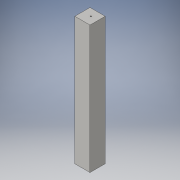
# Autodesk Inventor part: really cool squares
Saved by Autodesk Inventor 2016 (Build 200138000, 138)
## iProperties
Created: 2016-01-15
Part Number: really cool squares
Material: Generic
Document SubType Name: Modeling
Designer: Administrator
Density: 1 g/cm^3
Appearance: Default
Author: Administrator
Autodesk Inventor part; units mm, degrees
ref_plane "YZ Plane" through (0, 0, 0) normal (1, 0, 0) x (0, 1, 0)
ref_plane "XZ Plane" through (0, 0, 0) normal (0, 1, 0) x (-1, 0, 0)
ref_plane "XY Plane" through (0, 0, 0) normal (0, 0, 1) x (1, 0, 0)
sketch "Sketch1" plane through (0, 0, 0) normal (0, 1, 0) x (-1, 0, 0)
  line L0 (0, 0) -> (6.0452, 0)
  line L1 (6.0452, 0) -> (6.0452, 6.0452)
  line L2 (6.0452, 6.0452) -> (0, 6.0452)
  line L3 (0, 6.0452) -> (0, 0)
  dimension "d0" = 6.0452
  dimension "d1" = 6.0452
  constraints: 8 end point, 2 parallel, 1 horizontal, 1 perpendicular
  measures "d0" distance of L2.end L1.end
  measures "d1" distance of L1.end L0.end
extrude "Extrusion1" add sketch "Sketch1" along normal blind 50.8
hole "Hole1" at (-2.802, 50.8, 2.8898) direction (0, -1, 0) diameter 0.508 end through all
body "Solid1"
